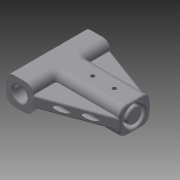
# Autodesk Inventor part: WagonAttachementV08
Saved by Autodesk Inventor 2014 (Build 180170000, 170)
## iProperties
Created: 2013-11-15
Part Number: WagonAttachementV08
Material: Generic
Document SubType Name: Modeling
Designer: steele
Density: 1 g/cm^3
Appearance: Default
Author: steele
Autodesk Inventor part; units mm, degrees
sketch "Base for Part" plane through (0, 0, 0) normal (0, 0, 1) x (1, 0, 0)
  line L0 (0, 0) -> (148, 0) construction
  line L1 (0, 0) -> (0, 50.8)
  line L2 (0, 50.8) -> (44.45, 50.8)
  line L3 (148, -29.2) -> (148, 0)
  line L4 (44.45, 50.8) -> (44.45, 25.4)
  line L5 (44.45, 25.4) -> (148, 25.4)
  line L6 (148, 25.4) -> (148, 0)
  line L7 (0, 0) -> (0, -50.8)
  line L8 (0, -50.8) -> (44.45, -50.8)
  line L9 (44.45, -50.8) -> (44.45, -25.4)
  line L10 (44.45, -25.4) -> (148, -25.4)
  line L11 (148, -25.4) -> (148, 0)
  dimension "d0" = 148
  dimension "d1" = 50.8
  dimension "d2" = 44.45
  dimension "d3" = 25.4
  constraints: 24 end point, 4 perpendicular, 4 symmetric about line, 2 parallel
  measures "d0" distance of L0.start L0.end
  measures "d1" distance of L0.start L1.end
  measures "d2" distance of L1.end L2.end
  measures "d3" distance of L2.end L4.end
extrude "Extrusion of Base" add sketch "Base for Part" along normal blind 44.45
sketch "Sketch for 1 inch PVC" plane through (148, -25.4, 0) normal (1, 0, 0) x (0, 0, -1)
  line L0 (0, 50.8) -> (-44.45, 50.8) projected
  line L1 (-44.45, 0) -> (-44.45, 50.8) projected
  line L2 (0, 0) -> (-44.45, 0) projected
  line L3 (-44.45, 25.4) -> (0, 25.4) construction
  line L4 (-22.225, 50.8) -> (-22.225, 0) construction
  circle A0 centre (-22.225, 25.4) radius 12.6619
  circle A1 centre (-22.225, 25.4) radius 17.0434
  dimension "d6" = 34.0868
  dimension "d7" = 25.3238
  constraints: 4 end point, 4 midpoint, 2 centre point, 1 coincident, 1 parallel
  measures "d6" diameter of A1
  measures "d7" diameter of A0
extrude "Extrusion for 1 inch PVC" cut sketch "Sketch for 1 inch PVC" against normal blind 114.55
sketch "Sketch of Base Hole" plane through (0, -50.8, 0) normal (0, -1, 0) x (1, 0, 0)
  line L0 (44.45, 0) -> (0, 0) projected
  line L1 (44.45, 0) -> (44.45, 44.45) projected
  line L2 (0, 44.45) -> (44.45, 44.45) projected
  line L3 (0, 0) -> (0, 44.45) projected
  line L4 (0, 22.225) -> (44.45, 22.225) construction
  line L5 (22.225, 44.45) -> (22.225, 0) construction
  circle A0 centre (22.225, 22.225) radius 11.1506
  dimension "d10" = 22.3012
  constraints: 5 midpoint, 4 end point, 1 centre point
  measures "d10" diameter of A0
extrude "Extrusion3" cut sketch "Sketch of Base Hole" against normal through all contours A0
ref_plane "Work Plane2" through (0, -44.45, 38.1) normal (-1, 0, 0) x (0, 0, 1)
sketch "Sketch5" plane through (0, -44.45, 38.1) normal (-1, 0, 0) x (0, 0, 1)
  line L0 (0, 0) -> (-31.75, 0) projected
  line L1 (-31.75, 88.9) -> (0, 88.9) projected
  line L2 (-31.75, 0) -> (-31.75, 88.9) projected
  line L3 (-18.75, 88.9) -> (-18.75, 0) construction
  line L4 (-8.75, 67.1607) -> (-18.75, 69.6729)
  line L5 (-18.75, 69.6729) -> (-18.75, 71.1639)
  line L6 (-18.75, 71.1639) -> (-10.4518, 73.198)
  line L7 (-10.4518, 73.198) -> (-18.75, 75.1753)
  line L8 (-18.75, 75.1753) -> (-18.75, 76.6502)
  line L9 (-18.75, 76.6502) -> (-8.75, 79.2028)
  line L10 (-8.75, 79.2028) -> (-8.75, 77.8333)
  line L11 (-8.75, 77.8333) -> (-17.0401, 75.8236)
  line L12 (-17.0401, 75.8236) -> (-8.75, 73.8301)
  line L13 (-8.75, 73.8301) -> (-8.75, 72.4767)
  line L14 (-8.75, 72.4767) -> (-17.1374, 70.467)
  line L15 (-17.1374, 70.467) -> (-8.75, 68.4654)
  line L16 (-8.75, 68.4654) -> (-8.75, 67.1607)
  spline S0 degree 2 poles (-17.9558, 61.8852) (-18.0693, 62.0391) (-18.4745, 62.5578) (-18.596, 62.8009) knots 0 0 0 1 2 2 2
  spline S1 degree 2 poles (-18.596, 62.8009) (-18.7743, 63.1331) (-18.9607, 63.7571) (-18.9607, 64.3244) knots 0 0 0 1 2 2 2
  spline S2 degree 2 poles (-18.9607, 64.3244) (-18.9607, 64.7863) (-18.6122, 65.621) (-18.2962, 65.937) knots 0 0 0 1 2 2 2
  spline S3 degree 2 poles (-18.2962, 65.937) (-17.9882, 66.2369) (-17.0806, 66.6015) (-16.5782, 66.6015) knots 0 0 0 1 2 2 2
  spline S4 degree 2 poles (-16.5782, 66.6015) (-15.8002, 66.6015) (-14.6981, 65.9451) (-14.3821, 65.232) knots 0 0 0 1 2 2 2
  spline S5 degree 2 poles (-14.3821, 65.232) (-14.0904, 64.5999) (-13.8716, 62.8819) (-13.8148, 61.8852) knots 0 0 0 1 2 2 2
  line L17 (-13.8148, 61.8852) -> (-13.5717, 61.8852)
  spline S6 degree 2 poles (-13.5717, 61.8852) (-13.1341, 61.8852) (-12.5912, 62.1526) (-12.4372, 62.3957) knots 0 0 0 1 2 2 2
  spline S7 degree 2 poles (-12.4372, 62.3957) (-12.2832, 62.6388) (-12.186, 63.3357) (-12.186, 63.7085) knots 0 0 0 1 2 2 2
  spline S8 degree 2 poles (-12.186, 63.7085) (-12.186, 64.1461) (-12.4453, 65.3293) (-12.6965, 65.9208) knots 0 0 0 1 2 2 2
  line L18 (-12.6965, 65.9208) -> (-12.6965, 65.9938)
  line L19 (-12.6965, 65.9938) -> (-11.408, 65.9938)
  spline S9 degree 2 poles (-11.408, 65.9938) (-11.3108, 65.6453) (-11.0677, 64.3406) (-11.0677, 63.7004) knots 0 0 0 1 2 2 2
  spline S10 degree 2 poles (-11.0677, 63.7004) (-11.0677, 62.9224) (-11.3108, 61.8609) (-11.6268, 61.4395) knots 0 0 0 1 2 2 2
  spline S11 degree 2 poles (-11.6268, 61.4395) (-11.9348, 61.0262) (-12.9153, 60.621) (-13.6203, 60.621) knots 0 0 0 1 2 2 2
  line L20 (-13.6203, 60.621) -> (-18.75, 60.621)
  line L21 (-18.75, 60.621) -> (-18.75, 61.8852)
  line L22 (-18.75, 61.8852) -> (-17.9558, 61.8852)
  line L23 (-16.9024, 61.8852) -> (-14.8197, 61.8852)
  spline S12 degree 2 poles (-14.8197, 61.8852) (-14.8602, 62.339) (-14.998, 63.7085) (-15.1276, 64.138) knots 0 0 0 1 2 2 2
  spline S13 degree 2 poles (-15.1276, 64.138) (-15.2816, 64.6404) (-15.9218, 65.2968) (-16.4891, 65.2968) knots 0 0 0 1 2 2 2
  spline S14 degree 2 poles (-16.4891, 65.2968) (-17.1374, 65.2968) (-17.7938, 64.5675) (-17.7938, 63.8706) knots 0 0 0 1 2 2 2
  spline S15 degree 2 poles (-17.7938, 63.8706) (-17.7938, 63.279) (-17.2832, 62.3066) (-16.9024, 61.8852) knots 0 0 0 1 2 2 2
  spline S16 degree 2 poles (-19.9494, 58.5788) (-20.0061, 58.4492) (-20.1844, 57.9549) (-20.2573, 57.6388) knots 0 0 0 1 2 2 2
  spline S17 degree 2 poles (-20.2573, 57.6388) (-20.3464, 57.2904) (-20.4518, 56.6988) (-20.4518, 56.3503) knots 0 0 0 1 2 2 2
  spline S18 degree 2 poles (-20.4518, 56.3503) (-20.4518, 55.7669) (-20.1438, 54.9565) (-19.8683, 54.7296) knots 0 0 0 1 2 2 2
  spline S19 degree 2 poles (-19.8683, 54.7296) (-19.5928, 54.5108) (-18.8716, 54.3406) (-18.4096, 54.3406) knots 0 0 0 1 2 2 2
  line L24 (-18.4096, 54.3406) -> (-17.7532, 54.3406)
  spline S20 degree 2 poles (-17.7532, 54.3406) (-18.1989, 54.8511) (-18.6203, 55.8317) (-18.6203, 56.5691) knots 0 0 0 1 2 2 2
  spline S21 degree 2 poles (-18.6203, 56.5691) (-18.6203, 57.8495) (-16.716, 59.3649) (-14.925, 59.3649) knots 0 0 0 1 2 2 2
  spline S22 degree 2 poles (-14.925, 59.3649) (-13.9931, 59.3649) (-12.5506, 58.8382) (-12.0401, 58.4006) knots 0 0 0 1 2 2 2
  spline S23 degree 2 poles (-12.0401, 58.4006) (-11.562, 57.9792) (-11.0353, 56.8203) (-11.0353, 56.2045) knots 0 0 0 1 2 2 2
  spline S24 degree 2 poles (-11.0353, 56.2045) (-11.0353, 55.621) (-11.3108, 54.7701) (-11.562, 54.3406) knots 0 0 0 1 2 2 2
  line L25 (-11.562, 54.3406) -> (-11.2459, 54.2677)
  line L26 (-11.2459, 54.2677) -> (-11.2459, 53.0764)
  line L27 (-11.2459, 53.0764) -> (-17.891, 53.0764)
  spline S25 degree 2 poles (-17.891, 53.0764) (-19.8035, 53.0764) (-21.5863, 54.7377) (-21.5863, 56.4476) knots 0 0 0 1 2 2 2
  spline S26 degree 2 poles (-21.5863, 56.4476) (-21.5863, 56.9986) (-21.408, 58.1494) (-21.2622, 58.6437) knots 0 0 0 1 2 2 2
  line L28 (-21.2622, 58.6437) -> (-19.9494, 58.6437)
  line L29 (-19.9494, 58.6437) -> (-19.9494, 58.5788)
  line L30 (-16.716, 54.3406) -> (-12.5912, 54.3406)
  spline S27 degree 2 poles (-12.5912, 54.3406) (-12.3643, 54.8106) (-12.1698, 55.6048) (-12.1698, 56.0019) knots 0 0 0 1 2 2 2
  spline S28 degree 2 poles (-12.1698, 56.0019) (-12.1698, 56.9581) (-13.5798, 58.0602) (-14.9007, 58.0602) knots 0 0 0 1 2 2 2
  spline S29 degree 2 poles (-14.9007, 58.0602) (-16.1487, 58.0602) (-17.4534, 57.2255) (-17.4534, 56.2855) knots 0 0 0 1 2 2 2
  spline S30 degree 2 poles (-17.4534, 56.2855) (-17.4534, 55.7912) (-17.0644, 54.7539) (-16.716, 54.3406) knots 0 0 0 1 2 2 2
  spline S31 degree 2 poles (-14.998, 45.078) (-16.8942, 45.078) (-18.9607, 46.9014) (-18.9607, 48.4249) knots 0 0 0 1 2 2 2
  spline S32 degree 2 poles (-18.9607, 48.4249) (-18.9607, 49.9889) (-16.8294, 51.7798) (-14.998, 51.7798) knots 0 0 0 1 2 2 2
  spline S33 degree 2 poles (-14.998, 51.7798) (-13.1179, 51.7798) (-11.0353, 49.9322) (-11.0353, 48.4249) knots 0 0 0 1 2 2 2
  spline S34 degree 2 poles (-11.0353, 48.4249) (-11.0353, 46.9014) (-13.1098, 45.078) (-14.998, 45.078) knots 0 0 0 1 2 2 2
  spline S35 degree 2 poles (-14.998, 46.3827) (-13.5393, 46.3827) (-12.1212, 47.4443) (-12.1212, 48.4249) knots 0 0 0 1 2 2 2
  spline S36 degree 2 poles (-12.1212, 48.4249) (-12.1212, 49.4054) (-13.5393, 50.4751) (-14.998, 50.4751) knots 0 0 0 1 2 2 2
  spline S37 degree 2 poles (-14.998, 50.4751) (-16.4161, 50.4751) (-17.8748, 49.4054) (-17.8748, 48.4249) knots 0 0 0 1 2 2 2
  spline S38 degree 2 poles (-17.8748, 48.4249) (-17.8748, 47.4524) (-16.4404, 46.3827) (-14.998, 46.3827) knots 0 0 0 1 2 2 2
  line L31 (-18.75, 37.89) -> (-18.75, 39.1542)
  line L32 (-18.75, 39.1542) -> (-14.4712, 39.1542)
  spline S39 degree 2 poles (-14.4712, 39.1542) (-13.9526, 39.1542) (-13.0612, 39.2515) (-12.7938, 39.3973) knots 0 0 0 1 2 2 2
  spline S40 degree 2 poles (-12.7938, 39.3973) (-12.5101, 39.5513) (-12.2346, 40.1024) (-12.2346, 40.5724) knots 0 0 0 1 2 2 2
  spline S41 degree 2 poles (-12.2346, 40.5724) (-12.2346, 41.0424) (-12.737, 42.0391) (-13.1422, 42.5173) knots 0 0 0 1 2 2 2
  line L33 (-13.1422, 42.5173) -> (-18.75, 42.5173)
  line L34 (-18.75, 42.5173) -> (-18.75, 43.7814)
  line L35 (-18.75, 43.7814) -> (-11.2459, 43.7814)
  line L36 (-11.2459, 43.7814) -> (-11.2459, 42.5173)
  line L37 (-11.2459, 42.5173) -> (-12.0806, 42.5173)
  spline S42 degree 2 poles (-12.0806, 42.5173) (-11.5701, 41.95) (-11.0353, 40.856) (-11.0353, 40.2401) knots 0 0 0 1 2 2 2
  spline S43 degree 2 poles (-11.0353, 40.2401) (-11.0353, 39.138) (-12.4939, 37.89) (-13.8797, 37.89) knots 0 0 0 1 2 2 2
  line L38 (-13.8797, 37.89) -> (-18.75, 37.89)
  line L39 (-8.75, 24.4703) -> (-18.75, 27.9143)
  line L40 (-18.75, 27.9143) -> (-18.75, 29.3487)
  line L41 (-18.75, 29.3487) -> (-8.75, 32.7928)
  line L42 (-8.75, 32.7928) -> (-8.75, 31.3665)
  line L43 (-8.75, 31.3665) -> (-17.0563, 28.5951)
  line L44 (-17.0563, 28.5951) -> (-8.75, 25.8236)
  line L45 (-8.75, 25.8236) -> (-8.75, 24.4703)
  spline S44 degree 2 poles (-13.75, 17.4605) (-16.4404, 17.4605) (-18.9607, 19.0246) (-18.9607, 20.6534) knots 0 0 0 1 2 2 2
  spline S45 degree 2 poles (-18.9607, 20.6534) (-18.9607, 22.3066) (-16.3918, 23.8544) (-13.7581, 23.8544) knots 0 0 0 1 2 2 2
  spline S46 degree 2 poles (-13.7581, 23.8544) (-11.0515, 23.8544) (-8.5474, 22.2904) (-8.5474, 20.6534) knots 0 0 0 1 2 2 2
  spline S47 degree 2 poles (-8.5474, 20.6534) (-8.5474, 19.0083) (-11.1406, 17.4605) (-13.75, 17.4605) knots 0 0 0 1 2 2 2
  spline S48 degree 2 poles (-16.797, 19.1785) (-16.3027, 18.984) (-14.7792, 18.822) (-13.75, 18.822) knots 0 0 0 1 2 2 2
  spline S49 degree 2 poles (-13.75, 18.822) (-12.7208, 18.822) (-11.2054, 18.984) (-10.6949, 19.1866) knots 0 0 0 1 2 2 2
  spline S50 degree 2 poles (-10.6949, 19.1866) (-10.1844, 19.3892) (-9.6576, 20.0942) (-9.6576, 20.6534) knots 0 0 0 1 2 2 2
  spline S51 degree 2 poles (-9.6576, 20.6534) (-9.6576, 21.2126) (-10.1844, 21.9338) (-10.7111, 22.1445) knots 0 0 0 1 2 2 2
  spline S52 degree 2 poles (-10.7111, 22.1445) (-11.2216, 22.3471) (-12.7776, 22.493) (-13.7581, 22.493) knots 0 0 0 1 2 2 2
  spline S53 degree 2 poles (-13.7581, 22.493) (-14.8116, 22.493) (-16.2216, 22.3633) (-16.7727, 22.1526) knots 0 0 0 1 2 2 2
  spline S54 degree 2 poles (-16.7727, 22.1526) (-17.2913, 21.9581) (-17.8505, 21.2369) (-17.8505, 20.6534) knots 0 0 0 1 2 2 2
  spline S55 degree 2 poles (-17.8505, 20.6534) (-17.8505, 20.1024) (-17.3237, 19.3811) (-16.797, 19.1785) knots 0 0 0 1 2 2 2
  spline S56 degree 2 poles (-18.9769, 13.1575) (-18.9769, 13.903) (-18.5312, 15.1267) (-18.1179, 15.5562) knots 0 0 0 1 2 2 2
  spline S57 degree 2 poles (-18.1179, 15.5562) (-17.7127, 15.9776) (-16.6106, 16.4152) (-15.9866, 16.4152) knots 0 0 0 1 2 2 2
  spline S58 degree 2 poles (-15.9866, 16.4152) (-15.1763, 16.4152) (-13.8148, 15.5481) (-13.4096, 14.7215) knots 0 0 0 1 2 2 2
  line L46 (-13.4096, 14.7215) -> (-13.3691, 14.7215)
  spline S59 degree 2 poles (-13.3691, 14.7215) (-12.9396, 15.4589) (-11.9186, 16.172) (-11.1568, 16.172) knots 0 0 0 1 2 2 2
  spline S60 degree 2 poles (-11.1568, 16.172) (-10.0304, 16.172) (-8.5231, 14.4703) (-8.5231, 13.1575) knots 0 0 0 1 2 2 2
  spline S61 degree 2 poles (-8.5231, 13.1575) (-8.5231, 11.796) (-9.9494, 10.151) (-11.0677, 10.151) knots 0 0 0 1 2 2 2
  spline S62 degree 2 poles (-11.0677, 10.151) (-11.7403, 10.151) (-13.0531, 10.937) (-13.4259, 11.6745) knots 0 0 0 1 2 2 2
  line L47 (-13.4259, 11.6745) -> (-13.4664, 11.6745)
  spline S63 degree 2 poles (-13.4664, 11.6745) (-13.8716, 10.7993) (-15.0385, 9.8998) (-15.9623, 9.8998) knots 0 0 0 1 2 2 2
  spline S64 degree 2 poles (-15.9623, 9.8998) (-17.2427, 9.8998) (-18.9769, 11.7636) (-18.9769, 13.1575) knots 0 0 0 1 2 2 2
  spline S65 degree 2 poles (-16.092, 11.2774) (-15.4761, 11.2774) (-14.7468, 11.7636) (-14.374, 12.4524) knots 0 0 0 1 2 2 2
  spline S66 degree 2 poles (-14.374, 12.4524) (-14.2443, 12.6793) (-13.9445, 13.4411) (-13.75, 13.9192) knots 0 0 0 1 2 2 2
  spline S67 degree 2 poles (-13.75, 13.9192) (-14.1147, 14.4703) (-15.2006, 15.0618) (-15.8894, 15.0618) knots 0 0 0 1 2 2 2
  spline S68 degree 2 poles (-15.8894, 15.0618) (-16.797, 15.0618) (-17.9801, 13.9678) (-17.9801, 13.1412) knots 0 0 0 1 2 2 2
  spline S69 degree 2 poles (-17.9801, 13.1412) (-17.9801, 12.2985) (-16.9672, 11.2774) (-16.092, 11.2774) knots 0 0 0 1 2 2 2
  spline S70 degree 2 poles (-11.0839, 11.4638) (-10.4113, 11.4638) (-9.5118, 12.3633) (-9.5118, 13.1656) knots 0 0 0 1 2 2 2
  spline S71 degree 2 poles (-9.5118, 13.1656) (-9.5118, 13.8949) (-10.314, 14.8268) (-11.0028, 14.8268) knots 0 0 0 1 2 2 2
  spline S72 degree 2 poles (-11.0028, 14.8268) (-11.4972, 14.8268) (-12.186, 14.3487) (-12.4615, 13.8706) knots 0 0 0 1 2 2 2
  spline S73 degree 2 poles (-12.4615, 13.8706) (-12.575, 13.668) (-12.972, 12.809) (-13.0855, 12.4605) knots 0 0 0 1 2 2 2
  spline S74 degree 2 poles (-13.0855, 12.4605) (-12.6398, 11.8771) (-11.6917, 11.4638) (-11.0839, 11.4638) knots 0 0 0 1 2 2 2
  point P0 (-38.1, 44.45)
  dimension "d25" = 13
  constraints: 2 end point, 2 point on line, 1 perpendicular, 1 vertical
  measures "d25" distance between parallel lines of L2 L3
emboss "Emboss1" sketch "Sketch5" operation cut depth 2 direction (1, 0, 0)
ref_plane "Work Plane1" through (0, 0, 44.45) normal (0, 0, 1) x (1, 0, 0)
sketch "Sketch9" plane through (0, 0, 44.45) normal (0, 0, 1) x (1, 0, 0)
  circle A0 centre (78.74, 0) radius 3.302
  circle A1 centre (114.3, 0) radius 3.302
  line L0 (149.86, 19.05) -> (149.86, -19.05) projected
  point P0 (0, 0)
  dimension "d39" = 6.604
  dimension "d42" = 35.56
  dimension "d43" = 71.12
  constraints: 2 centre point, 1 equal radius
  measures "d39" diameter of A0
  measures "d42" distance from line of A1.centre L0
  measures "d43" distance from line of L0 A0.centre
extrude "Extrusion6" cut sketch "Sketch9" against normal through all
sketch "Sketch10" plane through (0, 50.8, 0) normal (0, 1, 0) x (1, 0, 0)
  circle A0 centre (22.225, -22.225) radius 11.1506 projected
  line L0 (0, 0) -> (44.45, 0) projected
  line L1 (0, 0) -> (0, -44.45) projected
  line L2 (44.45, -44.45) -> (0, -44.45) projected
  line L3 (44.45, 0) -> (44.45, -44.45) projected
  circle A1 centre (22.225, -22.225) radius 11.1506
  line L4 (0, -44.45) -> (44.45, -44.45)
  line L5 (44.45, -44.45) -> (44.45, 0)
  line L6 (44.45, 0) -> (0, 0)
  line L7 (0, 0) -> (0, -44.45)
  line L8 (0, -44.45) -> (44.45, 0) construction
  line L9 (44.45, -44.45) -> (0, 0) construction
  constraints: 12 end point, 2 midpoint, 2 parallel, 1 centre point, 1 coincident, 1 concentric, 1 perpendicular
extrude "Extrusion7" add sketch "Sketch10" along normal blind 12.7
sketch "Sketch11" plane through (0, -50.8, 0) normal (0, -1, 0) x (1, 0, 0)
  circle A0 centre (22.225, 22.225) radius 11.1506 projected
  line L0 (44.45, 0) -> (0, 0) projected
  line L1 (44.45, 0) -> (44.45, 44.45) projected
  line L2 (0, 44.45) -> (44.45, 44.45) projected
  line L3 (0, 0) -> (0, 44.45) projected
  circle A1 centre (22.225, 22.225) radius 11.1506
  line L4 (0, 0) -> (44.45, 0)
  line L5 (44.45, 0) -> (44.45, 44.45)
  line L6 (44.45, 44.45) -> (0, 44.45)
  line L7 (0, 44.45) -> (0, 0)
  line L8 (0, 0) -> (44.45, 44.45) construction
  line L9 (44.45, 0) -> (0, 44.45) construction
  constraints: 12 end point, 2 midpoint, 2 parallel, 1 centre point, 1 coincident, 1 concentric, 1 perpendicular
extrude "Extrusion8" add sketch "Sketch11" along normal blind 12.7
sketch "Sketch15" plane through (44.45, -25.4, 0) normal (0, -1, 0) x (1, 0, 0)
  line L0 (103.55, 0) -> (0, 0) projected
  line L1 (103.55, 0) -> (103.55, 44.45) projected
  line L2 (0, 44.45) -> (103.55, 44.45) projected
  line L3 (0, 0) -> (0, 44.45) projected
  line L4 (0, 22.225) -> (103.55, 22.225) construction
  point P0 (-44.45, 0)
  constraints: 2 end point, 2 midpoint
sketch "Sketch16" plane through (44.45, -25.4, 44.45) normal (1, 0, 0) x (0, 0, -1)
  line L0 (44.45, 0) -> (44.45, -38.1) projected
  line L1 (44.45, 0) -> (0, 0) projected
  line L2 (0, 0) -> (0, -38.1) projected
  line L3 (44.45, -38.1) -> (0, -38.1) projected
  line L4 (22.225, 0) -> (22.225, -38.1) construction
  point P0 (44.45, 25.4)
  constraints: 2 end point, 2 midpoint
ref_plane "Work Plane6" through (44.45, -63.5, 22.225) normal (0, 0, -1) x (0, 1, 0)
ref_plane "Work Plane5" through (44.45, -63.5, 22.225) normal (0, 0, -1) x (0, 1, 0)
sketch "Sketch18" plane through (44.45, -25.4, 44.45) normal (1, 0, 0) x (0, 0, -1)
  line L0 (44.45, 0) -> (44.45, -38.1) projected
  line L1 (44.45, 0) -> (0, 0) projected
  line L2 (0, 0) -> (0, -38.1) projected
  line L3 (44.45, -38.1) -> (0, -38.1) projected
  point P0 (44.45, 25.4)
sketch "Sketch19" plane through (44.45, -63.5, 22.225) normal (0, 0, -1) x (0, 1, 0)
  line L0 (38, 104) -> (0, 0)
  line L1 (0, 0) -> (38, 0)
  line L2 (38, 0) -> (38, 104)
  point P0 (63.5, -44.45)
  constraints: 6 end point, 1 horizontal, 1 perpendicular
extrude "Extrusion9" add sketch "Sketch19" along normal mid plane 19.05
sketch "Sketch20" plane through (44.45, 25.4, 0) normal (0, 1, 0) x (1, 0, 0)
  line L0 (0, 0) -> (103.55, 0) projected
  line L1 (0, 0) -> (0, -44.45) projected
  line L2 (103.55, -44.45) -> (0, -44.45) projected
  line L3 (103.55, 0) -> (103.55, -44.45) projected
  line L4 (0, -22.225) -> (103.55, -22.225) construction
  point P0 (-44.45, 0)
  constraints: 2 end point, 2 midpoint
sketch "Sketch21" plane through (44.45, 25.4, 44.45) normal (1, 0, 0) x (0, 0, -1)
  line L0 (44.45, 38.1) -> (44.45, 0) projected
  line L1 (0, 38.1) -> (44.45, 38.1) projected
  line L2 (0, 0) -> (0, 38.1) projected
  line L3 (44.45, 0) -> (0, 0) projected
  line L4 (22.225, 38.1) -> (22.225, 0) construction
  point P0 (44.45, -25.4)
  constraints: 2 end point, 2 midpoint
ref_plane "Work Plane8" through (148, 25.4, 22.225) normal (0, 0, -1) x (-1, 0, 0)
ref_plane "Work Plane7" through (148, 25.4, 22.225) normal (0, 0, -1) x (-1, 0, 0)
sketch "Sketch29" plane through (148, -25.4, 0) normal (1, 0, 0) x (0, 0, -1)
  line L0 (0, 50.8) -> (0, 0) projected
  line L1 (-12.7, 50.8) -> (-31.75, 50.8) projected
  line L2 (-44.45, 0) -> (-44.45, 50.8) projected
  line L3 (0, 0) -> (-44.45, 0) projected
  line L4 (-44.45, 50.8) -> (0, 0) construction
  line L5 (-44.45, 0) -> (0, 50.8) construction
  line L6 (-44.45, 8) -> (0, 8) construction
  line L7 (-44.45, 43.8) -> (0, 43.8) construction
  circle A0 centre (-38.325, 43.8) radius 4
  circle A1 centre (-6.125, 43.8) radius 4
  circle A2 centre (-37.45, 8) radius 4
  circle A3 centre (-7, 8) radius 4
  point P0 (0, 25.4)
  dimension "d69" = 7
  dimension "d70" = 8
  dimension "d71" = 8
  constraints: 12 point on line, 8 end point, 4 centre point, 3 equal radius, 2 perpendicular
  measures "d69" distance between parallel lines of L1 L7
  measures "d70" distance between parallel lines of L3 L6
  measures "d71" diameter of A0
extrude "Extrusion13" cut sketch "Sketch29" against normal blind 143
sketch "Sketch32" plane through (148, -25.4, 0) normal (1, 0, 0) x (0, 0, -1)
  circle A0 centre (-37.45, 8) radius 4 projected
  circle A1 centre (-38.325, 43.8) radius 4 projected
  circle A2 centre (-6.125, 43.8) radius 4 projected
  circle A3 centre (-7, 8) radius 4 projected
  circle A4 centre (-38.325, 43.8) radius 4
  circle A5 centre (-6.125, 43.8) radius 4
  circle A6 centre (-7, 8) radius 4
  circle A7 centre (-37.45, 8) radius 4
  point P0 (0, 25.4)
  constraints: 4 centre point, 4 coincident, 4 concentric
extrude "Extrusion16" add sketch "Sketch32" against normal blind 5
sketch "Sketch33" plane through (148, -25.4, 0) normal (1, 0, 0) x (0, 0, -1)
  line L0 (0, 0) -> (-44.45, 0) projected
  circle A0 centre (-22.225, 25.4) radius 17.0434 projected
  line L1 (-22.225, 86.6) -> (-22.225, -39.4) construction
  circle A1 centre (-22.225, 63.5) radius 4
  circle A2 centre (-22.225, 76.2) radius 4
  circle A3 centre (-22.225, -12.7) radius 4
  circle A4 centre (-22.225, -25.4) radius 4
  point P0 (0, 25.4)
  dimension "d80" = 38.1
  dimension "d81" = 38.1
  dimension "d82" = 8
  dimension "d83" = 50.8
  dimension "d84" = 50.8
  constraints: 4 centre point, 4 point on line, 3 equal radius, 2 end point, 1 perpendicular
  measures "d80" distance of A3.centre A0.centre
  measures "d81" distance of A1.centre A0.centre
  measures "d82" diameter of A3
  measures "d83" distance of A2.centre A0.centre
  measures "d84" distance of A4.centre A0.centre
extrude "Extrusion17" cut sketch "Sketch33" against normal blind 114.55 contours A1 | A2 | A3 | A4
sketch "Sketch34" plane through (44.45, 25.4, 44.45) normal (1, 0, 0) x (0, 0, -1)
  circle A0 centre (22.225, 12.7) radius 4 projected
  circle A1 centre (22.225, 25.4) radius 4 projected
  line L0 (44.45, 38.1) -> (44.45, 0) projected
  line L1 (0, 38.1) -> (44.45, 38.1) projected
  line L2 (0, 0) -> (0, 38.1) projected
  line L3 (44.45, 0) -> (0, 0) projected
  line L4 (22.225, 38.1) -> (22.225, 0) construction
  point P0 (44.45, -25.4)
  constraints: 2 end point, 2 midpoint
sketch "Sketch35" plane through (44.45, 25.4, 0) normal (0, 1, 0) x (1, 0, 0)
  line L0 (0, 0) -> (103.55, 0) projected
  line L1 (0, 0) -> (0, -44.45) projected
  line L2 (103.55, -44.45) -> (0, -44.45) projected
  line L3 (103.55, 0) -> (103.55, -44.45) projected
  line L4 (0, -22.225) -> (103.55, -22.225) construction
  point P0 (-44.45, 0)
  constraints: 2 end point, 2 midpoint
ref_plane "Work Plane15" through (44.45, 63.5, 22.225) normal (0, 0, 1) x (0, -1, 0)
sketch "Sketch36" plane through (44.45, 63.5, 22.225) normal (0, 0, 1) x (0, -1, 0)
  line L0 (0, 0) -> (38, 103)
  line L1 (38, 103) -> (38, 0)
  line L2 (38, 0) -> (0, 0)
  point P0 (63.5, -44.45)
  constraints: 6 end point, 1 perpendicular, 1 vertical
extrude "Extrusion18" add sketch "Sketch36" along normal mid plane 19.05
sketch "Sketch37" plane through (148, -25.4, 0) normal (1, 0, 0) x (0, 0, -1)
  line L0 (0, 0) -> (-44.45, 0) projected
  circle A0 centre (-22.225, 25.4) radius 17.0434 projected
  line L1 (-22.225, 89.4818) -> (-22.225, 25.4) construction
  circle A1 centre (-22.225, 76.2) radius 4
  circle A2 centre (-22.225, 63.5) radius 4
  point P0 (0, 25.4)
  dimension "d89" = 8
  dimension "d90" = 38.1
  dimension "d91" = 50.8
  constraints: 2 centre point, 2 end point, 2 point on line, 1 equal radius, 1 perpendicular
  measures "d89" diameter of A2
  measures "d90" distance of L1.end A2.centre
  measures "d91" distance of L1.end A1.centre
extrude "Extrusion20" cut sketch "Sketch37" against normal blind 114.55 contours A1 | A2
fillet "Fillet25" radius 3.175 4 edges at (96.45, -44.5, 31.75) (96.45, -44.5, 12.7) (95.95, 44.5, 31.75) (95.95, 44.5, 12.7)
fillet "Fillet27" radius 3.175 2 edges at (44.45, 25.4, 22.225) (44.45, -25.4, 22.225)
fillet "Fillet28" radius 12.7 12 edges at (45.3799, -26.3299, 44.45) (44.45, -46.0375, 44.45) (97.8125, -25.4, 44.45) (45.3799, 26.3299, 44.45) (44.45, 46.0375, 44.45) (97.8125, 25.4, 44.45) (45.3799, -26.3299, 0) (44.45, -46.0375, 0) (97.8125, -25.4, 0) (45.3799, 26.3299, 0) (44.45, 46.0375, 0) (97.8125, 25.4, 0)
fillet "Fillet29" radius 12.7 2 edges at (0, 0, 0) (0, 0, 44.45)
fillet "Fillet30" radius 3.175 4 edges at (11.0744, 63.5, 22.225) (148, 0, 34.8869) (148, 0, 39.2684) (11.0744, -63.5, 22.225)
fillet "Fillet31" radius 3.175 8 edges at (148, 0, 0) (148, -21.6803, 3.7197) (148, -25.4, 22.225) (148, -21.6803, 40.7303) (148, 0, 44.45) (148, 21.6803, 40.7303) (148, 25.4, 22.225) (148, 21.6803, 3.7197)
sketch "Sketch38" plane through (148, 0, 22.225) normal (1, 0, 0) x (0, 0, -1)
  circle A0 centre (0, 0) radius 9.4869 projected
  circle A1 centre (0, 0) radius 5
  point P0 (22.225, 0)
  dimension "d112" = 10
  constraints: 1 centre point, 1 coincident
  measures "d112" diameter of A1
extrude "Extrusion21" cut sketch "Sketch38" against normal blind 114.55 contours A1
sketch "Sketch39" plane through (148, 0, 22.225) normal (1, 0, 0) x (0, 0, -1)
  circle A0 centre (0, 0) radius 5 projected
  circle A1 centre (0, 0) radius 9.4869 projected
  circle A2 centre (0, 0) radius 5
  point P0 (22.225, 0)
  constraints: 1 centre point, 1 coincident, 1 concentric
extrude "Extrusion22" add sketch "Sketch39" against normal blind 5 contours A0
body "Solid1"
